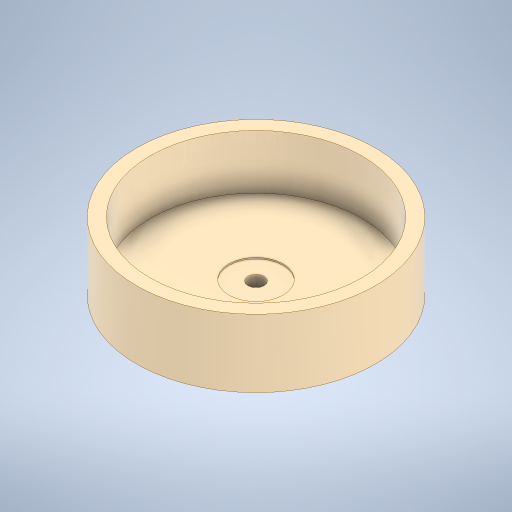
# Autodesk Inventor part: bottom
Saved by Autodesk Inventor 2024 (Build 280153020, 153B)
## iProperties
Created: 2023-06-12
Part Number: bottom
Material: Polyethylene, High Density
Document SubType Name: Modeling
Designer: OKESH
Density: 0.952 g/cm^3
Appearance: Smooth - Off-White
Author: OKESH
Autodesk Inventor part; units mm, degrees
ref_plane "YZ Plane" through (0, 0, 0) normal (1, 0, 0) x (0, 1, 0)
ref_plane "XZ Plane" through (0, 0, 0) normal (0, 1, 0) x (-1, 0, 0)
ref_plane "XY Plane" through (0, 0, 0) normal (0, 0, 1) x (1, 0, 0)
sketch "Sketch1" plane through (0, 0, 0) normal (0, 1, 0) x (-1, 0, 0)
  circle A0 centre (0, 0) radius 44
  dimension "d0" = 88
  constraints: 1 centre point, 1 coincident
  measures "d0" diameter of A0
extrude "Extrusion1" add sketch "Sketch1" along normal blind 25
sketch "Sketch2" plane through (0, 25, 0) normal (0, 1, 0) x (1, 0, 0)
  circle A0 centre (0, 0) radius 44
  circle A1 centre (0, 0) radius 39
  dimension "d5" = 5
  constraints: 2 centre point, 1 coincident
  measures "d5" radial gap between concentric circles of A0 A1
extrude "Extrusion2" cut sketch "Sketch2" against normal blind 20 contours A1
sketch "Sketch3" plane through (0, 0, 0) normal (0, -1, 0) x (1, 0, 0)
  circle A0 centre (0, 0) radius 3
  circle A1 centre (0, 0) radius 5
  dimension "d8" = 6
  dimension "d9" = 2
  constraints: 2 centre point, 1 coincident
  measures "d8" diameter of A0
  measures "d9" radial gap between concentric circles of A0 A1
extrude "Extrusion3" cut sketch "Sketch3" against normal blind 20 contours A0
extrude "Extrusion4" cut sketch "Sketch3" against normal blind 0.5
fillet "Fillet1" radius 0.2 1 edges at (-5, 0, 0)
sketch "Sketch4" plane through (0, 5, 0) normal (0, 1, 0) x (1, 0, 0)
  circle A0 centre (0, 0) radius 3 projected
  circle A1 centre (0, 0) radius 10
  dimension "d15" = 20
  constraints: 1 centre point, 1 coincident
  measures "d15" diameter of A1
extrude "Extrusion5" cut sketch "Sketch4" against normal blind 0.5
body "Solid1"
